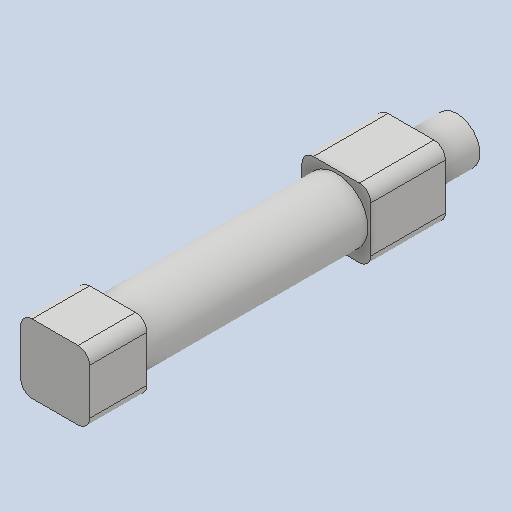
# Autodesk Inventor part: summer_cilinder
Saved by Autodesk Inventor 2024.1 (Build 281209000, 209)
## iProperties
Created: 2019-08-21
Part Number: summer_cilinder
Material: 一般
Document SubType Name: Modeling
Designer: Haruka
Density: 1 g/cm^3
Appearance: 既定
Mass: 7.15295 g
Surface Area: 31.3453 cm^2
Volume: 7.15295 cm^3
Author: Haruka
Autodesk Inventor part; units mm, degrees
ref_plane "YZ Plane" through (0, 0, 0) normal (1, 0, 0) x (0, 1, 0)
ref_plane "XZ Plane" through (0, 0, 0) normal (0, 1, 0) x (-1, 0, 0)
ref_plane "XY Plane" through (0, 0, 0) normal (0, 0, 1) x (1, 0, 0)
sketch "スケッチ1" plane through (0, 0, 0) normal (0, 1, 0) x (-1, 0, 0)
  line L0 (0, 0) -> (12, 0)
  line L1 (12, 0) -> (12, -12)
  line L2 (12, -12) -> (0, -12)
  line L3 (0, -12) -> (0, 0)
  dimension "d0" = 12
  dimension "d1" = 12
  constraints: 8 end point, 2 parallel, 1 horizontal, 1 perpendicular
  measures "d0" distance of L1.end L2.end
  measures "d1" distance of L0.end L1.end
extrude "押し出し1" add sketch "スケッチ1" along normal blind 10
sketch "スケッチ2" plane through (0, 10, 0) normal (0, 1, 0) x (1, 0, 0)
  line L0 (-12, 0) -> (0, 0) projected
  line L1 (-6, 0) -> (-6, 12)
  line L2 (0, 12) -> (-12, 12) projected
  line L3 (-12, 12) -> (-12, 0) projected
  line L4 (-12, 6) -> (0, 6)
  circle A0 centre (-6, 6) radius 5.5
  dimension "d4" = 11
  constraints: 4 end point, 4 midpoint, 1 centre point, 1 horizontal
  measures "d4" diameter of A0
extrude "押し出し2" add sketch "スケッチ2" along normal blind 39 contours A0 L4 L1 | L1 L4 A0 | A0 L1 L4 | L1 A0 L4
sketch "スケッチ3" plane through (-6, 49, -6) normal (0, 1, 0) x (1, 0, 0)
  line L0 (-6, 6) -> (-6, -6) projected
  line L1 (6, -6) -> (6, 6) projected
  line L2 (-6, 6) -> (6, 6)
  line L3 (6, 6) -> (6, -6)
  line L4 (6, -6) -> (-6, -6)
  line L5 (-6, -6) -> (-6, 6)
  constraints: 8 end point, 2 parallel, 1 horizontal, 1 perpendicular
extrude "押し出し3" add sketch "スケッチ3" along normal blind 13
fillet "フィレット1" radius 2 8 edges at (0, 55.5, 0) (0, 5, 0) (0, 5, -12) (0, 55.5, -12) (-12, 55.5, 0) (-12, 5, 0) (-12, 5, -12) (-12, 55.5, -12)
sketch "スケッチ4" plane through (-6, 62, -6) normal (0, 1, 0) x (1, 0, 0)
  circle A0 centre (0, 0) radius 4
  point P0 (6, -6)
  dimension "d10" = 8
  constraints: 1 centre point
  measures "d10" diameter of A0
extrude "押し出し4" add sketch "スケッチ4" along normal blind 8
sketch "スケッチ5" plane through (-6, 70, -6) normal (0, 1, 0) x (1, 0, 0)
  circle A0 centre (0, 0) radius 2
  point P0 (6, -6)
  dimension "d13" = 4
  constraints: 1 centre point
  measures "d13" diameter of A0
extrude "押し出し5" cut sketch "スケッチ5" against normal blind 15
